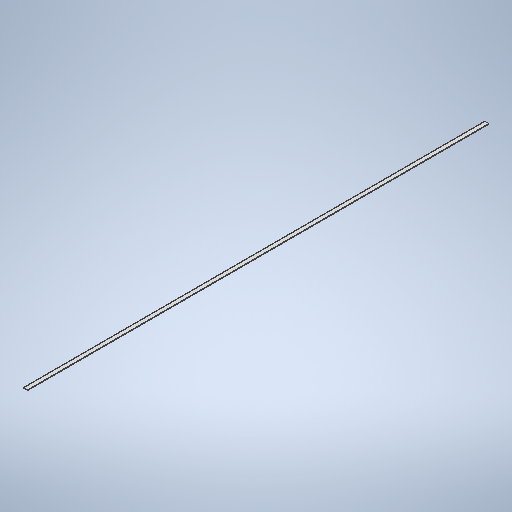
# Autodesk Inventor part: HD - 404 PERFIL DE ALUMINIO - CLIP DE TRAVESAÑO HORIZONTAL
Saved by Autodesk Inventor 2025 (Build 290162000, 162)
## iProperties
Created: 2026-01-25
Part Number: HD - 404 PERFIL DE ALUMINIO - CLIP DE TRAVESAÑO HORIZONTAL
Material: Generic
Document SubType Name: Modeling
Designer: Frank
Density: 1 g/cm^3
Appearance: Default
Author: Frank
Autodesk Inventor part; units mm, degrees
ref_plane "YZ Plane" through (0, 0, 0) normal (1, 0, 0) x (0, 1, 0)
ref_plane "XZ Plane" through (0, 0, 0) normal (0, 1, 0) x (-1, 0, 0)
ref_plane "XY Plane" through (0, 0, 0) normal (0, 0, 1) x (1, 0, 0)
sketch "Sketch1" plane through (0, 0, 0) normal (0, 0, 1) x (1, 0, 0)
  line L0 (-22.2, 8.1341) -> (0.1434, 8.1341)
  line L1 (-0.5, 0) -> (-1.5, 0)
  line L2 (-2, 0.5) -> (-2, 5.8341)
  line L3 (-2.5, 6.3341) -> (-22.2, 6.3341)
  line L4 (0.1806, 5.0309) -> (0.5561, 4.6085)
  line L5 (0.0723, 5.4961) -> (0.6254, 7.5011)
  line L6 (0.6112, 4.0192) -> (0.0712, 3.1187)
  line L7 (0, 0.5) -> (0, 2.8616)
  line L8 (-22.2, 15.4691) -> (-22.2, -2.8641) construction
  arc A0 (-2, 5.8341) -> (-2.5, 6.3341) centre (-2.5, 5.8341) ccw
  arc A1 (0.6254, 7.5011) -> (0.1434, 8.1341) centre (0.1434, 7.6341) ccw
  arc A2 (0.0723, 5.4961) -> (0.1806, 5.0309) centre (0.5543, 5.3631) ccw
  arc A3 (0.6112, 4.0192) -> (0.5561, 4.6085) centre (0.1824, 4.2763) ccw
  arc A4 (0.0712, 3.1187) -> (0, 2.8616) centre (0.5, 2.8616) ccw
  arc A5 (-0.5, 0) -> (0, 0.5) centre (-0.5, 0.5) ccw
  arc A6 (-2, 0.5) -> (-1.5, 0) centre (-1.5, 0.5) ccw
  line L9 (-22.2, 8.1341) -> (-44.5434, 8.1341)
  line L10 (-43.9, 0) -> (-42.9, 0)
  line L11 (-42.4, 0.5) -> (-42.4, 5.8341)
  line L12 (-41.9, 6.3341) -> (-22.2, 6.3341)
  line L13 (-44.5806, 5.0309) -> (-44.9561, 4.6085)
  line L14 (-44.4723, 5.4961) -> (-45.0254, 7.5011)
  line L15 (-45.0112, 4.0192) -> (-44.4712, 3.1187)
  line L16 (-44.4, 0.5) -> (-44.4, 2.8616)
  arc A7 (-41.9, 6.3341) -> (-42.4, 5.8341) centre (-41.9, 5.8341) ccw
  arc A8 (-44.5434, 8.1341) -> (-45.0254, 7.5011) centre (-44.5434, 7.6341) ccw
  arc A9 (-44.5806, 5.0309) -> (-44.4723, 5.4961) centre (-44.9543, 5.3631) ccw
  arc A10 (-44.9561, 4.6085) -> (-45.0112, 4.0192) centre (-44.5824, 4.2763) ccw
  arc A11 (-44.4, 2.8616) -> (-44.4712, 3.1187) centre (-44.9, 2.8616) ccw
  arc A12 (-44.4, 0.5) -> (-43.9, 0) centre (-43.9, 0.5) ccw
  arc A13 (-42.9, 0) -> (-42.4, 0.5) centre (-42.9, 0.5) ccw
  point P0 (0, 0)
  point P1 (0, 0)
  point P2 (0, 5.2341)
  point P3 (0.8, 8.1341)
  point P4 (0, 3)
  point P5 (0.8, 4.3341)
  point P6 (-44.4, 0)
  point P7 (-44.4, 0)
  point P8 (-44.4, 5.2341)
  point P9 (-45.2, 8.1341)
  point P10 (-44.4, 3)
  point P11 (-45.2, 4.3341)
  dimension "d7" = 0.8
  dimension "d8" = 0.8
  dimension "d9" = 3.8
  dimension "d10" = 2.9
  dimension "d12" = 3
  dimension "d13" = 8.1341
  dimension "d14" = 2.2341
  dimension "d15" = 1.8
  dimension "d16" = 2
  dimension "d18" = 0.5
  dimension "d19" = 46
  constraints: 34 end point, 28 point on circle, 27 symmetric about line, 22 point on line, 14 centre point, 14 tangent, 6 equal radius, 2 coincident, 1 horizontal, 1 perpendicular, 1 vertical, 7 other
  measures "d7" distance from line of L7 point (0.8, 4.334)
  measures "d8" distance from line of L7 point (0.8, 8.134)
  measures "d9" distance of point (0.8, 4.334) point (0.8, 8.134)
  measures "d10" distance from line of point (0, 5.234) L0
  measures "d12" distance from line of L1 point (0, 3)
  measures "d13" distance between parallel lines of L1 L0
  measures "d14" distance of point (0, 3) point (0, 5.234)
  measures "d15" distance between parallel lines of L0 L3
  measures "d16" distance between parallel lines of L7 L2
  measures "d18" radius of A0
  measures "d19" distance of point (0.8, 8.134) point (-45.2, 8.134)
extrude "Extrusion1" add sketch "Sketch1" against normal blind 5000
body "Solid1"
